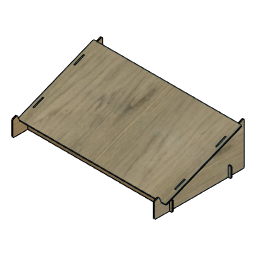
laptop stand v4 (Autodesk Fusion 360 design; units mm, degrees)
Autodesk Fusion 360 part; units mm, degrees
note: some values were not read from the file. Chosen so that the rebuilt part matches the saved one: that a step has no effect.
sketch "Sketch1" plane through (0, 0, 0) normal (1, 0, 0) x (0, 1, 0)
  line L0 (0, 0) -> (260, 0)
  line L1 (260, 0) -> (260, 125)
  line L2 (260, 125) -> (21.6995, 28.7203)
  line L3 (21.6995, 28.7203) -> (13, 50.2523)
  line L4 (13, 50.2523) -> (0, 45)
  line L5 (0, 45) -> (0, 0)
  dimension "d1" = 260
  dimension "d2" = 125
  dimension "d3" = 45
  dimension "d4" = 22
  dimension "d5" = 13
  constraint coincident L0.start L5.end
  constraint horizontal L0
  constraint perpendicular L0 L1
  constraint perpendicular L2 L3
  constraint parallel L2 L4
  constraint vertical L5
  measures "d1" distance of L0.start L0.end
  measures "d2" distance of L0.end L1.end
  measures "d3" vertical distance of L4.end L0.start
  measures "d4" angle of L0 L2
  measures "d5" distance of L3.end L5
extrude "Extrude1" add sketch "Sketch1" along normal blind 3 makes body 1
fillet "Fillet1" radius 3 4 edges at (1.5, 260, 125) (1.5, 13, 50.2523) (1.5, 0, 45) (1.5, 21.6995, 28.7203) on bodies 1
fillet "Fillet2" radius 3 2 edges at (1.5, 0, 0) (1.5, 260, 0) on bodies 1
move_face "MoveFace1" [no effect]
copy_body "CopyPasteBodies1" bodies 1 makes body 2
move_body "Move1" bodies 2 to x (1, 0, 0) y (0, 1, 0) z (0, 0, 1) at (410, 0, 0)
sketch "Sketch2" plane through (0, -6.9303, 17.1531) normal (0, -0.374607, 0.927184) x (1, 0, 0) in component "top"
  line L0 (410, 33.8782) -> (413, 33.8782)
  line L1 (413, 33.8782) -> (413, 283.4459)
  line L2 (413, 283.4459) -> (410, 283.4459)
  line L3 (410, 283.4459) -> (410, 33.8782)
  line L4 (-8, 271.4459) -> (421, 271.4459)
  line L5 (421, 271.4459) -> (421, 33.8782)
  line L6 (421, 33.8782) -> (-8, 33.8782)
  line L7 (-8, 33.8782) -> (-8, 271.4459)
  line L8 (0, 33.8782) -> (3, 33.8782)
  line L9 (3, 33.8782) -> (3, 283.4459)
  line L10 (3, 283.4459) -> (0, 283.4459)
  line L11 (0, 283.4459) -> (0, 33.8782)
  line L12 (410, 231.4459) -> (413, 231.4459)
  line L13 (413, 231.4459) -> (413, 201.4459)
  line L14 (413, 201.4459) -> (410, 201.4459)
  line L15 (410, 201.4459) -> (410, 231.4459)
  line L16 (206.5, 271.4459) -> (206.5, 33.8782) construction
  line L17 (-8, 152.6621) -> (421, 152.6621) construction
  line L18 (410, 73.8782) -> (413, 73.8782)
  line L19 (413, 103.8782) -> (410, 103.8782)
  line L20 (3, 231.4459) -> (0, 231.4459)
  line L21 (0, 201.4459) -> (3, 201.4459)
  line L22 (3, 73.8782) -> (0, 73.8782)
  line L23 (0, 103.8782) -> (3, 103.8782)
  dimension "d14" = 12
  dimension "d15" = 8
  dimension "d16" = 8
  dimension "d17" = 30
  dimension "d18" = 40
  constraint horizontal L4
  constraint vertical L5
  constraint horizontal L6
  constraint vertical L7
  constraint collinear L6 L8
  constraint horizontal L12
  constraint vertical L13
  constraint horizontal L14
  constraint vertical L15
  constraint coincident L1 L13.end
  constraint coincident L3 L12.start
  constraint midpoint L4 L16.start
  constraint midpoint L6 L16.end
  constraint midpoint L7 L17.start
  constraint midpoint L5 L17.end
  constraint symmetric L12.start L17 L18.start
  constraint symmetric L12.end L17 L18.end
  constraint symmetric L13.end L17 L19.start
  constraint symmetric L14.end L17 L19.end
  constraint symmetric L12.start L16 L20.start
  constraint symmetric L12.end L16 L20.end
  constraint symmetric L13.end L16 L21.start
  constraint symmetric L14.end L16 L21.end
  constraint symmetric L16 L18.start L22.start
  constraint symmetric L16 L18.end L22.end
  constraint symmetric L16 L19.start L23.start
  constraint symmetric L16 L19.end L23.end
  measures "d14" distance of L2 L4
  measures "d15" distance of L1 L5
  measures "d16" distance of L7 L11
  measures "d17" distance of L12 L14
  measures "d18" distance of L4 L12
extrude "Extrude1'" add sketch "Sketch2" against normal blind 3 separate body contours L0 L1 L3 L6 L18 | L3 L4 L6 L9 L15 | L1 L4 L5 L6 L13 | L6 L8 L9 L11 L22 | L1 L3 L14 L19 | L4 L6 L7 L11 | L9 L11 L21 L23 | L1 L3 L4 L12 | L4 L9 L11 L20 makes body 3 in component "top"
combine "Combine1" operation cut target body 2 tool bodies 3 keep tools
combine "Combine2" operation cut target body 1 tool bodies 3 keep tools
fillet "Fillet1'" radius 3 4 edges at (421, 25.043, 28.4534) (421, 245.3119, 117.4478) (-8, 245.3119, 117.4478) (-8, 25.043, 28.4534) on bodies 3 in component "top"
ref_plane "WorkPlane1" through (411.5, 215, 61.7762) normal (0, 1, 0) x (0, 0, 1) in component "support"
sketch "Sketch1 (2)" plane through (411.5, 215, 61.7762) normal (0, 1, 0) x (1, 0, 0) in component "support"
  line L0 (-1.5, -41.8071) -> (1.5, -41.8071)
  line L1 (1.5, -41.8071) -> (1.5, 61.7762)
  line L2 (1.5, 61.7762) -> (-1.5, 61.7762)
  line L3 (-1.5, 61.7762) -> (-1.5, -41.8071)
  line L4 (-411.5, -41.8071) -> (-408.5, -41.8071)
  line L5 (-408.5, -41.8071) -> (-408.5, 61.7762)
  line L6 (-408.5, 61.7762) -> (-411.5, 61.7762)
  line L7 (-411.5, 61.7762) -> (-411.5, -41.8071)
  line L8 (9.5, 61.7762) -> (-419.5, 61.7762)
  line L9 (-419.5, 61.7762) -> (-419.5, 31.7762)
  line L10 (-419.5, 31.7762) -> (9.5, 31.7762)
  line L11 (9.5, 31.7762) -> (9.5, 61.7762)
  line L12 (-419.5, 33.5897) -> (-419.5, -53.1571)
  line L13 (9.5, -53.1571) -> (9.5, 33.5897)
  line L14 (9.5, 46.7762) -> (-419.5, 46.7762)
  dimension "d24" = 30
  constraint horizontal L8
  constraint vertical L9
  constraint horizontal L10
  constraint vertical L11
  constraint collinear L6 L8
  constraint collinear L9 L12
  constraint collinear L11 L13
  constraint midpoint L11 L14.start
  constraint midpoint L9 L14.end
  measures "d24" distance of L8 L10
extrude "Extrude1''" add sketch "Sketch1 (2)" along normal mid plane 3 separate body contours L3 L5 L10 L14 | L1 L10 L11 L13 L14 | L3 L5 L8 L14 | L1 L2 L3 L8 L14 | L1 L8 L11 L14 | L5 L6 L7 L8 L14 | L7 L9 L10 L12 L14 | L7 L8 L9 L14 makes body 4 in component "support"
ref_plane "WorkPlane2" through (411.5, 130, 61.7762) normal (0, 1, 0) x (0, 0, 1) in component "support"
fillet "Fillet1''" radius 2 4 edges at (-8, 215, 30) (-8, 215, 0) (421, 215, 30) (421, 215, 0) on bodies 4 in component "support"
fillet "Fillet2'" radius 0.5 4 edges at (410, 215, 30) (413, 215, 30) (0, 215, 30) (3, 215, 30) on bodies 4 in component "support"
mirror "Mirror1" about plane through (411.5, 130, 61.7762) normal (0, 1, 0) of bodies 4 makes body 5 in component "support"
combine "Combine3" operation cut target body 2 tool bodies 4 keep tools
combine "Combine4" operation cut target body 2 tool bodies 5 keep tools
combine "Combine5" operation cut target body 1 tool bodies 4 keep tools
combine "Combine6" operation cut target body 1 tool bodies 5 keep tools
fillet "Fillet3" radius 0.5 8 edges at (1.5, 43.5, 0) (1.5, 46.5, 0) (1.5, 213.5, 0) (1.5, 216.5, 0) (411.5, 213.5, 0) (411.5, 216.5, 0) (411.5, 46.5, 0) (411.5, 43.5, 0) on bodies 1 2
fillet "Fillet4" radius 0.5 8 edges at (1.5, 207.6626, 103.8543) (1.5, 179.8471, 92.6161) (1.5, 89.3839, 56.0666) (1.5, 61.5684, 44.8284) (411.5, 61.5684, 44.8284) (411.5, 89.3839, 56.0666) (411.5, 207.6626, 103.8543) (411.5, 179.8471, 92.6161) on bodies 1 2
sketch "leg.DXF" plane through (413, 0, 0) normal (1, 0, 0) x (0, 1, 0)
  arc A0 (180.3107, 92.8034) -> (180.0344, 92.1525) centre (180.498, 92.3398) ccw
  line L0 (180.0344, 92.1525) -> (180.9709, 89.8346)
  line L1 (180.9709, 89.8346) -> (90.5077, 53.2851)
  line L2 (90.5077, 53.2851) -> (89.5712, 55.603)
  arc A1 (89.5712, 55.603) -> (88.9203, 55.8793) centre (89.1076, 55.4157) ccw
  line L3 (88.9203, 55.8793) -> (62.032, 45.0157)
  arc A2 (62.032, 45.0157) -> (61.7557, 44.3648) centre (62.2193, 44.5521) ccw
  line L4 (61.7557, 44.3648) -> (62.6922, 42.0469)
  line L5 (62.6922, 42.0469) -> (25.6049, 27.0626)
  line L6 (25.6049, 27.0626) -> (24.481, 29.8442)
  arc A3 (20.5757, 31.5019) -> (24.481, 29.8442) centre (23.3572, 32.6257) ccw
  line L7 (20.5757, 31.5019) -> (14.1238, 47.4708)
  arc A4 (14.1238, 47.4708) -> (10.2184, 49.1285) centre (11.3423, 46.347) ccw
  line L8 (10.2184, 49.1285) -> (1.8762, 45.758)
  arc A5 (1.8762, 45.758) -> (0, 42.9765) centre (3, 42.9765) ccw
  line L9 (0, 42.9765) -> (0, 3)
  arc A6 (0, 3) -> (3, 0) centre (3, 3) ccw
  line L10 (3, 0) -> (43, 0)
  arc A7 (43, 0) -> (43.5, 0.5) centre (43, 0.5) ccw
  line L11 (43.5, 0.5) -> (43.5, 15)
  line L12 (43.5, 15) -> (46.5, 15)
  line L13 (46.5, 15) -> (46.5, 0.5)
  arc A8 (46.5, 0.5) -> (47, 0) centre (47, 0.5) ccw
  line L14 (47, 0) -> (213, 0)
  arc A9 (213, 0) -> (213.5, 0.5) centre (213, 0.5) ccw
  line L15 (213.5, 0.5) -> (213.5, 15)
  line L16 (213.5, 15) -> (216.5, 15)
  line L17 (216.5, 15) -> (216.5, 0.5)
  arc A10 (216.5, 0.5) -> (217, 0) centre (217, 0.5) ccw
  line L18 (217, 0) -> (257, 0)
  arc A11 (257, 0) -> (260, 3) centre (257, 3) ccw
  line L19 (260, 3) -> (260, 120.5523)
  arc A12 (260, 120.5523) -> (255.8762, 123.3339) centre (257, 120.5523) ccw
  line L20 (255.8762, 123.3339) -> (244.75, 118.8386)
  line L21 (244.75, 118.8386) -> (245.8738, 116.057)
  line L22 (245.8738, 116.057) -> (208.7864, 101.0728)
  line L23 (208.7864, 101.0728) -> (207.8499, 103.3907)
  arc A13 (207.8499, 103.3907) -> (207.199, 103.667) centre (207.3863, 103.2034) ccw
  line L24 (207.199, 103.667) -> (180.3107, 92.8034)
sketch "support.DXF" plane through (0, 213.5, 0) normal (0, -1, 0) x (1, 0, 0)
  arc A0 (3.5, 30) -> (3, 29.5) centre (3.5, 29.5) ccw
  line L0 (3, 29.5) -> (3, 15)
  line L1 (3, 15) -> (0, 15)
  line L2 (0, 15) -> (0, 29.5)
  arc A1 (0, 29.5) -> (-0.5, 30) centre (-0.5, 29.5) ccw
  line L3 (-0.5, 30) -> (-6, 30)
  arc A2 (-6, 30) -> (-8, 28) centre (-6, 28) ccw
  line L4 (-8, 28) -> (-8, 2)
  arc A3 (-8, 2) -> (-6, 0) centre (-6, 2) ccw
  line L5 (-6, 0) -> (419, 0)
  arc A4 (419, 0) -> (421, 2) centre (419, 2) ccw
  line L6 (421, 2) -> (421, 28)
  arc A5 (421, 28) -> (419, 30) centre (419, 28) ccw
  line L7 (419, 30) -> (413.5, 30)
  arc A6 (413.5, 30) -> (413, 29.5) centre (413.5, 29.5) ccw
  line L8 (413, 29.5) -> (413, 15)
  line L9 (413, 15) -> (410, 15)
  line L10 (410, 15) -> (410, 29.5)
  arc A7 (410, 29.5) -> (409.5, 30) centre (409.5, 29.5) ccw
  line L11 (409.5, 30) -> (3.5, 30)
sketch "top.DXF" plane through (0, -6.9303, 17.1531) normal (0, -0.374607, 0.927184) x (1, 0, 0)
  arc A0 (-8, 36.8782) -> (-5, 33.8782) centre (-5, 36.8782) ccw
  line L0 (-5, 33.8782) -> (418, 33.8782)
  arc A1 (418, 33.8782) -> (421, 36.8782) centre (418, 36.8782) ccw
  line L1 (421, 36.8782) -> (421, 268.4459)
  arc A2 (421, 268.4459) -> (418, 271.4459) centre (418, 268.4459) ccw
  line L2 (418, 271.4459) -> (-5, 271.4459)
  arc A3 (-5, 271.4459) -> (-8, 268.4459) centre (-5, 268.4459) ccw
  line L3 (-8, 268.4459) -> (-8, 36.8782)
  line L4 (410, 103.8782) -> (413, 103.8782)
  line L5 (413, 103.8782) -> (413, 73.8782)
  line L6 (413, 73.8782) -> (410, 73.8782)
  line L7 (410, 73.8782) -> (410, 103.8782)
  line L8 (3, 103.8782) -> (3, 73.8782)
  line L9 (3, 73.8782) -> (0, 73.8782)
  line L10 (0, 73.8782) -> (0, 103.8782)
  line L11 (0, 103.8782) -> (3, 103.8782)
  line L12 (3, 201.4459) -> (0, 201.4459)
  line L13 (0, 201.4459) -> (0, 231.4459)
  line L14 (0, 231.4459) -> (3, 231.4459)
  line L15 (3, 231.4459) -> (3, 201.4459)
  line L16 (413, 201.4459) -> (410, 201.4459)
  line L17 (410, 201.4459) -> (410, 231.4459)
  line L18 (410, 231.4459) -> (413, 231.4459)
  line L19 (413, 231.4459) -> (413, 201.4459)
component "top" placed x (1, 0, 0) y (0, 1, 0) z (0, 0, 1) at (0, 0, 0)
component "support" placed x (1, 0, 0) y (0, 1, 0) z (0, 0, 1) at (0, 0, 0)
equation "thickness = 3 mm"
equation "legwidth = 410 mm"
equation "d8 = thickness"
equation "d19 = -thickness"
equation "d25 = thickness"
